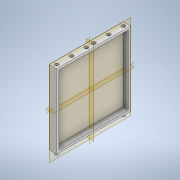
# Autodesk Inventor part: Wall
Saved by Autodesk Inventor 2022.4 (Build 264492010, 492A)
## iProperties
Created: 2025-02-20
Part Number: Wall
Material: Generic
Document SubType Name: Modeling
Designer: jan-m
Density: 1 g/cm^3
Appearance: Default
Author: jan-m
Autodesk Inventor part; units mm, degrees
sketch "Sketch2" plane through (0, 0, 0) normal (1, 0, 0) x (0, 1, 0)
  line L0 (49.875, 49.875) -> (-49.875, 49.875)
  line L1 (-49.875, 49.875) -> (-49.875, -49.875)
  line L2 (-49.875, -49.875) -> (49.875, -49.875)
  line L3 (49.875, -49.875) -> (49.875, 49.875)
  line L4 (-69.825, 0) -> (69.825, 0) projected
  line L5 (0, 69.825) -> (0, -69.825) projected
  point P0 (0, 0)
  point P1 (49.875, 0)
  point P2 (0, 49.875)
  dimension "d0" = 99.75
  dimension "d1" = 99.75
  constraints: 8 end point, 2 midpoint, 2 parallel, 2 point on line, 1 horizontal, 1 perpendicular
  measures "d0" distance of L2.end L0.start
  measures "d1" distance of L1.end L2.end
extrude "Extrusion1" add sketch "Sketch2" along normal mid plane 9.75
sketch "Sketch3" plane through (4.875, 0, 0) normal (1, 0, 0) x (0, 0, -1)
  line L0 (-46.875, 46.875) -> (46.875, 46.875)
  line L1 (46.875, 46.875) -> (46.875, -46.875)
  line L2 (46.875, -46.875) -> (-46.875, -46.875)
  line L3 (-46.875, -46.875) -> (-46.875, 46.875)
  line L4 (0, -69.825) -> (0, 69.825) projected
  line L5 (-69.825, 0) -> (69.825, 0) projected
  point P0 (0, 0)
  point P1 (0, 46.875)
  point P2 (-46.875, 0)
  dimension "d4" = 93.75
  dimension "d5" = 93.75
  constraints: 8 end point, 2 midpoint, 2 parallel, 2 point on line, 1 horizontal, 1 perpendicular
  measures "d4" distance of L0.start L0.end
  measures "d5" distance of L0.end L1.end
extrude "Extrusion2" cut sketch "Sketch3" against normal blind 7
sketch "Sketch5" plane through (-4.875, 49.875, 49.875) normal (0, 1, 0) x (1, 0, 0)
  circle A0 centre (4.875, 4.875) radius 2.5
  line L0 (9.75, 0) -> (0, 0) projected
  line L1 (4.875, 119.7) -> (4.875, -19.95) projected
  circle A1 centre (4.875, 24.875) radius 2.5
  circle A2 centre (4.875, 44.875) radius 2.5
  circle A3 centre (4.875, 94.875) radius 2.5
  line L2 (0, 99.75) -> (9.75, 99.75) projected
  circle A4 centre (4.875, 74.875) radius 2.5
  circle A5 centre (4.875, 54.875) radius 2.5
  point P0 (4.875, 49.875)
  dimension "d26" = 5
  dimension "d27" = 4.875
  dimension "d30" = 20
  dimension "d35" = 5
  dimension "d36" = 4.875
  dimension "d39" = 20
  constraints: 6 centre point, 2 point on line, 2 vertical, 8 other
  measures "d26" diameter of A0
  measures "d27" distance from line of L0 A0.centre
  measures "d30" distance of A0.centre A1.centre
  measures "d35" diameter of A3
  measures "d36" distance from line of L2 A3.centre
  measures "d39" distance of A3.centre A4.centre
extrude "Extrusion3" cut sketch "Sketch5" against normal blind 7
sketch "Sketch6" plane through (-4.875, -49.875, -49.875) normal (0, -1, 0) x (1, 0, 0)
  circle A0 centre (4.875, 94.875) radius 2.375
  line L0 (0, 99.75) -> (9.75, 99.75) projected
  line L1 (4.875, -19.95) -> (4.875, 119.7) projected
  line L2 (4.875, 119.7) -> (4.875, -19.95) projected
  line L3 (0, 0) -> (9.75, 0) projected
  line L4 (-1.95, 49.875) -> (11.7, 49.875) projected
  circle A1 centre (4.875, 4.875) radius 2.375
  point P0 (4.875, 49.875)
  dimension "d46" = 4.75
  dimension "d47" = 4.875
  constraints: 2 centre point, 1 point on line, 1 symmetric about line, 1 other
  measures "d46" diameter of A0
  measures "d47" distance from line of L0 A0.centre
extrude "Extrusion4" add sketch "Sketch6" along normal blind 4.75
body "Solid1"
